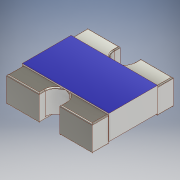
# Autodesk Inventor part: ResistorArray-1632
Saved by Autodesk Inventor 2018 (Build 220112000, 112)
## iProperties
Created: 2018-09-29
Part Number: ResistorArray-1632
Material: Copper
Document SubType Name: Modeling
Designer: Bradley
Density: 8.94 g/cm^3
Appearance: Copper - Satin
Author: Bradley
Autodesk Inventor part; units mm, degrees
ref_plane "YZ Plane" through (0, 0, 0) normal (1, 0, 0) x (0, 1, 0)
ref_plane "XZ Plane" through (0, 0, 0) normal (0, 1, 0) x (-1, 0, 0)
ref_plane "XY Plane" through (0, 0, 0) normal (0, 0, 1) x (1, 0, 0)
sketch "Sketch1" plane through (0, 0, 0) normal (0, 0, 1) x (1, 0, 0)
  line L0 (-0.8, -0.45) -> (0.8, -0.45)
  line L1 (0.8, -0.45) -> (0.8, 0.45)
  line L2 (0.8, 0.45) -> (-0.8, 0.45)
  line L3 (-0.8, 0.45) -> (-0.8, -0.45)
  line L4 (-0.8, -0.45) -> (0.8, 0.45) construction
  line L5 (0.8, -0.45) -> (-0.8, 0.45) construction
  point P0 (0, 0)
  dimension "d0" = 1.6
  dimension "d1" = 0.9
  constraints: 12 end point, 2 midpoint, 2 parallel, 1 horizontal, 1 perpendicular
  measures "d0" distance of L2.end L1.end
  measures "d1" distance of L2.end L0.start
extrude "Extrusion1" add sketch "Sketch1" along normal mid plane 0.45
sketch "Sketch2" plane through (0, 0, 0) normal (0, 0, 1) x (1, 0, 0)
  line L0 (-0.8, -0.45) -> (0.8, -0.45) projected
  line L1 (0.8, -0.45) -> (0.8, 0.45) projected
  line L2 (0.8, 0.45) -> (-0.8, 0.45) projected
  line L3 (-0.8, 0.45) -> (-0.8, -0.45) projected
  line L4 (0.8, 0.45) -> (-0.8, 0.45) projected
  line L5 (-0.79, 0.45) -> (-0.19, 0.45)
  line L6 (-0.19, 0.45) -> (-0.19, 0.75)
  line L7 (-0.19, 0.75) -> (-0.79, 0.75)
  line L8 (-0.79, 0.75) -> (-0.79, 0.45)
  line L9 (0.79, -0.45) -> (0.19, -0.45)
  line L10 (0.19, -0.45) -> (0.19, -0.75)
  line L11 (0.19, -0.75) -> (0.79, -0.75)
  line L12 (0.79, -0.75) -> (0.79, -0.45)
  line L13 (0.79, 0.45) -> (0.19, 0.45)
  line L14 (0.19, 0.45) -> (0.19, 0.75)
  line L15 (0.19, 0.75) -> (0.79, 0.75)
  line L16 (0.79, 0.75) -> (0.79, 0.45)
  line L17 (-0.8, -0.45) -> (0.8, -0.45) projected
  line L18 (0.8, -0.45) -> (-0.8, -0.45) projected
  line L19 (-0.79, -0.45) -> (-0.19, -0.45)
  line L20 (-0.19, -0.45) -> (-0.19, -0.75)
  line L21 (-0.19, -0.75) -> (-0.79, -0.75)
  line L22 (-0.79, -0.75) -> (-0.79, -0.45)
  point P0 (0, 0)
  dimension "d4" = 0.6
  dimension "d18" = 0.01
  dimension "d19" = 0.01
  dimension "d26" = 1.5
  constraints: 32 end point, 8 collinear, 8 parallel, 4 horizontal, 4 perpendicular, 4 point on line
  measures "d4" distance of L6.end L7.end
  measures "d18" distance between parallel lines of L1 L16
  measures "d19" distance between parallel lines of L3 L8
  measures "d26" distance between parallel lines of L21 L7
extrude "Extrusion2" add sketch "Sketch2" along normal blind 0.2 and the other way blind 0.275 contours L0 L20 L21 L22 | L8 L7 L6 L2 | L0 L12 L11 L10 | L14 L15 L16 L2
fillet "Fillet2" radius 0.19 4 edges at (-0.19, -0.45, -0.0125) (0.19, -0.45, -0.0125) (-0.19, 0.45, -0.0125) (0.19, 0.45, -0.0125)
fillet "Fillet3" radius 0.02 28 edges at (-0.79, -0.6, 0.2) (-0.49, -0.75, 0.2) (-0.19, -0.6948, 0.2) (0.19, -0.6948, 0.2) (0.49, -0.75, 0.2) (0.79, -0.6, 0.2) (0.79, -0.6, -0.275) (0.49, -0.75, -0.275) (-0.19, -0.6, -0.275) (0.19, -0.6, -0.275) (-0.49, -0.75, -0.275) (0.79, 0.6, 0.2) (0.49, 0.75, 0.2) (0.19, 0.6947, 0.2) (-0.19, 0.6947, 0.2) (-0.79, 0.6, 0.2) (-0.49, 0.75, 0.2) (0.79, 0.6, -0.275) (0.49, 0.75, -0.275) (-0.19, 0.6, -0.275) (0.19, 0.6, -0.275) (-0.49, 0.75, -0.275) (-0.79, 0.6, -0.275) (-0.49, -0.45, -0.275) (-0.79, -0.6, -0.275) (0.49, -0.45, -0.275) (0.49, 0.45, -0.275) (-0.49, 0.45, -0.275)
equation "\"d19\" = d18"
body "Solid1"
